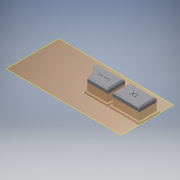
# Autodesk Inventor part: buttons
Saved by Autodesk Inventor 2017.3 (Build 213257000, 257)
## iProperties
Created: 2021-12-05
Part Number: buttons
Material: Generic
Document SubType Name: Modeling
Designer: TEOS
Density: 1 g/cm^3
Appearance: Default
Author: TEOS
Autodesk Inventor part; units mm, degrees
ref_plane "YZ Plane" through (0, 0, 0) normal (1, 0, 0) x (0, 1, 0)
ref_plane "XZ Plane" through (0, 0, 0) normal (0, 1, 0) x (-1, 0, 0)
ref_plane "XY Plane" through (0, 0, 0) normal (0, 0, 1) x (1, 0, 0)
ref_plane "Work Plane1" through (0, 0, 0) normal (0, 0, 1) x (1, 0, 0)
ref_plane "Work Plane2" through (0, 0, 0) normal (0, 0, 1) x (1, 0, 0)
sketch "Sketch3" plane through (0, 0, 0) normal (0, 0, 1) x (1, 0, 0)
  circle A0 centre (67, -22) radius 12.5 projected
  circle A1 centre (27, -22) radius 12.5 projected
  line L0 (-20.5, 34.5) -> (25.5, 34.5) projected
  line L1 (25.5, 34.5) -> (25.5, 4.5) projected
  line L2 (25.5, 4.5) -> (-9.3082, 4.5) projected
  arc A2 (-9.3082, 4.5) -> (-20.5, 25.0657) centre (-48.5, -3.5) ccw projected
  line L3 (-20.5, 25.0657) -> (-20.5, 34.5) projected
  line L4 (79.5, 4.5) -> (33.5, 4.5) projected
  line L5 (33.5, 4.5) -> (33.5, 34.5) projected
  line L6 (33.5, 34.5) -> (79.5, 34.5) projected
  line L7 (79.5, 34.5) -> (79.5, 4.5) projected
  circle A3 centre (-48.5, -3.5) radius 34 projected
  arc A4 (-82, 44) -> (-89, 37) centre (-82, 37) ccw projected
  line L8 (-89, -37) -> (-89, 37) projected
  arc A5 (-89, -37) -> (-82, -44) centre (-82, -37) ccw projected
  line L9 (82, -44) -> (-82, -44) projected
  arc A6 (82, -44) -> (89, -37) centre (82, -37) ccw projected
  line L10 (89, 37) -> (89, -37) projected
  arc A7 (89, 37) -> (82, 44) centre (82, 37) ccw projected
  line L11 (-82, 44) -> (82, 44) projected
  arc A8 (-9.064, 4.8) -> (-20.2, 25.1915) centre (-48.5, -3.5) ccw
  line L12 (-9.064, 4.8) -> (25.2, 4.8)
  line L13 (25.2, 4.8) -> (25.2, 34.2)
  line L14 (25.2, 34.2) -> (-20.2, 34.2)
  line L15 (-20.2, 34.2) -> (-20.2, 25.1915)
  line L16 (33.8, 34.2) -> (33.8, 4.8)
  line L17 (33.8, 4.8) -> (79.2, 4.8)
  line L18 (79.2, 4.8) -> (79.2, 34.2)
  line L19 (79.2, 34.2) -> (33.8, 34.2)
  point P0 (0, 0)
  dimension "d10" = 0.3
  dimension "d11" = 0.3
  constraints: 16 end point, 2 point on circle, 1 centre point, 7 other
  measures "d10" radial gap between concentric circles of A2 A8
  measures "d11" distance between parallel lines of L5 L16
extrude "Extrusion3" add sketch "Sketch3" along normal blind 7 and the other way blind 13 contours A8 L15 L14 L13 L12 | L19 L18 L17 L16
sketch "Sketch4" plane through (0, 0, -13) normal (0, 0, -1) x (-1, 0, 0)
  arc A0 (20.2, 25.1915) -> (9.064, 4.8) centre (48.5, -3.5) ccw projected
  line L0 (20.2, 25.1915) -> (20.2, 34.2) projected
  line L1 (20.2, 34.2) -> (-25.2, 34.2) projected
  line L2 (-25.2, 34.2) -> (-25.2, 4.8) projected
  line L3 (-25.2, 4.8) -> (9.064, 4.8) projected
  line L4 (-33.8, 4.8) -> (-33.8, 34.2) projected
  line L5 (-33.8, 34.2) -> (-79.2, 34.2) projected
  line L6 (-79.2, 34.2) -> (-79.2, 4.8) projected
  line L7 (-79.2, 4.8) -> (-33.8, 4.8) projected
  arc A1 (23.2, 23.908) -> (11.5785, 1.8) centre (48.5, -3.5) ccw
  line L8 (23.2, 23.908) -> (23.2, 37.2)
  line L9 (23.2, 37.2) -> (-28.2, 37.2)
  line L10 (-28.2, 37.2) -> (-28.2, 1.8)
  line L11 (-28.2, 1.8) -> (11.5785, 1.8)
  line L12 (-30.8, 37.2) -> (-30.8, 1.8)
  line L13 (-30.8, 1.8) -> (-82.2, 1.8)
  line L14 (-82.2, 1.8) -> (-82.2, 37.2)
  line L15 (-82.2, 37.2) -> (-30.8, 37.2)
  point P0 (0, 0)
  dimension "d16" = 3
  dimension "d17" = 3
  constraints: 16 end point, 2 point on circle, 1 centre point, 7 other
  measures "d16" radial gap between concentric circles of A0 A1
  measures "d17" distance between parallel lines of L4 L12
extrude "Extrusion4" add sketch "Sketch4" along normal blind 3 contours A0 L3 L2 L1 L0 | L7 L6 L5 L4 | A1 L11 L10 L9 L8 | L12 L13 L14 L15
sketch "Sketch5" plane through (0, 0, -16) normal (0, 0, -1) x (-1, 0, 0)
  arc A0 (23.2, 23.908) -> (11.5785, 1.8) centre (48.5, -3.5) ccw projected
  line L0 (23.2, 23.908) -> (23.2, 37.2) projected
  line L1 (23.2, 37.2) -> (-28.2, 37.2) projected
  line L2 (-28.2, 37.2) -> (-28.2, 1.8) projected
  line L3 (-28.2, 1.8) -> (11.5785, 1.8) projected
  line L4 (-30.8, 1.8) -> (-30.8, 37.2) projected
  line L5 (-30.8, 37.2) -> (-82.2, 37.2) projected
  line L6 (-82.2, 37.2) -> (-82.2, 1.8) projected
  line L7 (-82.2, 1.8) -> (-30.8, 1.8) projected
  line L8 (-82.2, 19.5) -> (15.4079, 19.5) construction
  arc A1 (20.2, 25.1915) -> (9.064, 4.8) centre (48.5, -3.5) ccw construction
  line L9 (-82.2, 37.2) -> (-30.8, 37.2) construction
  line L10 (-56.5, 37.2) -> (-56.5, 1.8) construction
  line L11 (-30.8, 1.8) -> (-82.2, 1.8) construction
  line L12 (23.2, 37.2) -> (-28.2, 37.2) construction
  line L13 (-2.5, 37.2) -> (-2.5, 1.8) construction
  line L14 (-28.2, 1.8) -> (11.5785, 1.8) construction
  point P0 (0, 0)
  point P1 (-16.2, 19.5)
  point P2 (5.2, 19.5)
  point P3 (-70.2, 19.5)
  point P4 (-42.8, 19.5)
  dimension "d20" = 12
  dimension "d21" = 18
  dimension "d22" = 12
  constraints: 6 end point, 5 point on line, 4 midpoint, 1 horizontal, 1 parallel, 1 point on circle, 1 symmetric about line
  measures "d20" distance from line of L2 point (-16.2, 19.5)
  measures "d21" distance from line of L0 point (5.2, 19.5)
  measures "d22" distance from line of L6 point (-70.2, 19.5)
hole "Hole1" at (16.2, 19.5, -16) at (-5.2, 19.5, -16) at (70.2, 19.5, -16) at (42.8, 19.5, -16) direction (0, 0, 1) diameter 5 depth 8
chamfer "Chamfer1" distance 2 angle 45 8 edges at (33.8, 19.5, 7) (56.5, 34.2, 7) (79.2, 19.5, 7) (56.5, 4.8, 7) (2.5, 34.2, 7) (25.2, 19.5, 7) (8.068, 4.8, 7) (-13.1306, 15.8157, 7)
sketch "Sketch6" plane through (0, 0, 7) normal (0, 0, 1) x (1, 0, 0)
  line L0 (62.1554, 16.2385) -> (50.9463, 16.2385) construction
  line L1 (50.9463, 16.2385) -> (50.9463, 23.2385) construction
  line L2 (50.9463, 23.2385) -> (62.1554, 23.2385) construction
  line L3 (62.1554, 23.2385) -> (62.1554, 16.2385) construction
  line L4 (77.2, 32.2) -> (77.2, 6.8) projected
  line L5 (35.8, 6.8) -> (35.8, 32.2) projected
  line L6 (77.2, 6.8) -> (35.8, 32.2)
  line L7 (77.2, 6.8) -> (35.8, 6.8) projected
  line L8 (35.8, 32.2) -> (35.8, 6.8)
  line L9 (35.8, 32.2) -> (77.2, 32.2) projected
  line L10 (35.8, 6.8) -> (77.2, 32.2)
  line L11 (59.8126, 23.2385) -> (59.8126, 17.0667)
  line L12 (59.8126, 17.0667) -> (62.1611, 17.0667)
  line L13 (62.1611, 17.0667) -> (62.1611, 16.2385)
  line L14 (62.1611, 16.2385) -> (56.5338, 16.2385)
  line L15 (56.5338, 16.2385) -> (56.5338, 17.0667)
  line L16 (56.5338, 17.0667) -> (58.8823, 17.0667)
  line L17 (58.8823, 17.0667) -> (58.8823, 23.2385)
  line L18 (58.8823, 23.2385) -> (59.8126, 23.2385)
  line L19 (50.986, 23.2385) -> (52.0525, 23.2385)
  line L20 (52.0525, 23.2385) -> (53.7542, 20.4476)
  line L21 (53.7542, 20.4476) -> (55.4901, 23.2385)
  line L22 (55.4901, 23.2385) -> (56.4941, 23.2385)
  line L23 (56.4941, 23.2385) -> (54.2648, 19.7328)
  line L24 (54.2648, 19.7328) -> (56.426, 16.2385)
  line L25 (56.426, 16.2385) -> (55.3596, 16.2385)
  line L26 (55.3596, 16.2385) -> (53.6919, 18.9784)
  line L27 (53.6919, 18.9784) -> (51.9901, 16.2385)
  line L28 (51.9901, 16.2385) -> (50.986, 16.2385)
  line L29 (50.986, 16.2385) -> (53.1756, 19.6875)
  line L30 (53.1756, 19.6875) -> (50.986, 23.2385)
  point P0 (0, 0)
  constraints: 6 end point, 1 perpendicular, 2 other
emboss "Emboss1" sketch "Sketch6" operation cut depth 25 direction (0, 0, -1) contours L11 L6 L17 L10 | L10 L17 L18 L11 | L14 L15 L16 L17 L6 L11 L12 | L6 L12 L13 L14 | L30 L19 L20 L6 | L6 L20 L21 L23 L24 L10 L26 L27 L28 L29 L30 | L10 L27 L28 | L21 L22 L23 L6 | L24 L25 L26 L10
sketch "Sketch7" plane through (0, 0, 7) normal (0, 0, 1) x (1, 0, 0)
  line L0 (14.8194, 18.056) -> (-5.029, 18.056) construction
  line L1 (-5.029, 18.056) -> (-5.029, 21.7006) construction
  line L2 (-5.029, 21.7006) -> (14.8194, 21.7006) construction
  line L3 (14.8194, 21.7006) -> (14.8194, 18.056) construction
  line L4 (23.2, 6.8) -> (-7.4732, 6.8) projected
  line L5 (-20.2, 32.2) -> (23.2, 32.2) projected
  line L6 (23.2, 6.8) -> (-20.2, 32.2)
  line L7 (23.2, 32.2) -> (23.2, 6.8) projected
  line L8 (-20.2, 32.2) -> (23.2, 32.2)
  line L9 (23.2, 32.2) -> (-20.2, 6.8)
  line L10 (13.648, 21.6269) -> (13.648, 18.541)
  line L11 (13.648, 18.541) -> (14.8223, 18.541)
  line L12 (14.8223, 18.541) -> (14.8223, 18.1269)
  line L13 (14.8223, 18.1269) -> (12.0087, 18.1269)
  line L14 (12.0087, 18.1269) -> (12.0087, 18.541)
  line L15 (12.0087, 18.541) -> (13.1829, 18.541)
  line L16 (13.1829, 18.541) -> (13.1829, 21.6269)
  line L17 (13.1829, 21.6269) -> (13.648, 21.6269)
  line L18 (9.646, 21.6269) -> (10.0885, 21.6269)
  line L19 (10.0885, 21.6269) -> (10.0885, 21.3376)
  spline S0 degree 2 poles (10.0885, 21.3376) (10.2927, 21.5163) (10.6586, 21.7006) (10.8855, 21.7006) knots 0 0 0 1 2 2 2
  spline S1 degree 2 poles (10.8855, 21.7006) (11.0557, 21.7006) (11.3591, 21.5872) (11.4698, 21.4652) knots 0 0 0 1 2 2 2
  spline S2 degree 2 poles (11.4698, 21.4652) (11.5832, 21.3433) (11.708, 20.9717) (11.708, 20.7051) knots 0 0 0 1 2 2 2
  line L20 (11.708, 20.7051) -> (11.708, 19.0005)
  line L21 (11.708, 19.0005) -> (11.2655, 19.0005)
  line L22 (11.2655, 19.0005) -> (11.2655, 20.4981)
  spline S3 degree 2 poles (11.2655, 20.4981) (11.2655, 20.7079) (11.2343, 20.9831) (11.1804, 21.0852) knots 0 0 0 1 2 2 2
  spline S4 degree 2 poles (11.1804, 21.0852) (11.1266, 21.1873) (10.9422, 21.2809) (10.7692, 21.2809) knots 0 0 0 1 2 2 2
  spline S5 degree 2 poles (10.7692, 21.2809) (10.6075, 21.2809) (10.2416, 21.0965) (10.0885, 20.9632) knots 0 0 0 1 2 2 2
  line L23 (10.0885, 20.9632) -> (10.0885, 19.0005)
  line L24 (10.0885, 19.0005) -> (9.646, 19.0005)
  line L25 (9.646, 19.0005) -> (9.646, 21.6269)
  line L26 (6.943, 21.6269) -> (7.3855, 21.6269)
  line L27 (7.3855, 21.6269) -> (7.3855, 20.1293)
  spline S6 degree 2 poles (7.3855, 20.1293) (7.3855, 19.9478) (7.4195, 19.6358) (7.4706, 19.5422) knots 0 0 0 1 2 2 2
  spline S7 degree 2 poles (7.4706, 19.5422) (7.5245, 19.4429) (7.7173, 19.3465) (7.8818, 19.3465) knots 0 0 0 1 2 2 2
  spline S8 degree 2 poles (7.8818, 19.3465) (8.0463, 19.3465) (8.3952, 19.5224) (8.5625, 19.6642) knots 0 0 0 1 2 2 2
  line L28 (8.5625, 19.6642) -> (8.5625, 21.6269)
  line L29 (8.5625, 21.6269) -> (9.005, 21.6269)
  line L30 (9.005, 21.6269) -> (9.005, 19.0005)
  line L31 (9.005, 19.0005) -> (8.5625, 19.0005)
  line L32 (8.5625, 19.0005) -> (8.5625, 19.2926)
  spline S9 degree 2 poles (8.5625, 19.2926) (8.364, 19.1139) (7.9811, 18.9267) (7.7655, 18.9267) knots 0 0 0 1 2 2 2
  spline S10 degree 2 poles (7.7655, 18.9267) (7.3798, 18.9267) (6.943, 19.4373) (6.943, 19.9223) knots 0 0 0 1 2 2 2
  line L33 (6.943, 19.9223) -> (6.943, 21.6269)
  spline S11 degree 2 poles (5.1817, 21.6865) (5.8113, 21.6865) (6.5034, 20.9802) (6.5034, 20.3279) knots 0 0 0 1 2 2 2
  spline S12 degree 2 poles (6.5034, 20.3279) (6.5034, 19.6869) (5.8312, 18.9267) (5.2894, 18.9267) knots 0 0 0 1 2 2 2
  spline S13 degree 2 poles (5.2894, 18.9267) (5.0455, 18.9267) (4.6683, 19.0686) (4.5293, 19.2189) knots 0 0 0 1 2 2 2
  spline S14 degree 2 poles (4.5293, 19.2189) (4.3875, 19.3692) (4.2372, 19.8032) (4.2372, 20.118) knots 0 0 0 1 2 2 2
  line L34 (4.2372, 20.118) -> (4.2372, 20.3591)
  line L35 (4.2372, 20.3591) -> (6.0552, 20.3591)
  spline S15 degree 2 poles (6.0552, 20.3591) (6.0552, 20.8157) (5.5958, 21.3007) (5.1873, 21.3007) knots 0 0 0 1 2 2 2
  spline S16 degree 2 poles (5.1873, 21.3007) (5.0427, 21.3007) (4.7619, 21.2355) (4.6484, 21.1844) knots 0 0 0 1 2 2 2
  spline S17 degree 2 poles (4.6484, 21.1844) (4.5293, 21.1277) (4.3648, 21.0284) (4.3109, 20.9831) knots 0 0 0 1 2 2 2
  line L36 (4.3109, 20.9831) -> (4.2854, 20.9831)
  line L37 (4.2854, 20.9831) -> (4.2854, 21.4652)
  spline S18 degree 2 poles (4.2854, 21.4652) (4.362, 21.4964) (4.5946, 21.5872) (4.6853, 21.6127) knots 0 0 0 1 2 2 2
  spline S19 degree 2 poles (4.6853, 21.6127) (4.8129, 21.6496) (5.0228, 21.6865) (5.1817, 21.6865) knots 0 0 0 1 2 2 2
  spline S20 degree 2 poles (4.6683, 20.0216) (4.674, 19.8429) (4.7477, 19.5819) (4.8186, 19.494) knots 0 0 0 1 2 2 2
  spline S21 degree 2 poles (4.8186, 19.494) (4.8952, 19.3947) (5.1363, 19.2898) (5.315, 19.2898) knots 0 0 0 1 2 2 2
  spline S22 degree 2 poles (5.315, 19.2898) (5.4908, 19.2898) (5.7376, 19.3947) (5.8397, 19.4968) knots 0 0 0 1 2 2 2
  spline S23 degree 2 poles (5.8397, 19.4968) (5.939, 19.6018) (6.0411, 19.8542) (6.0552, 20.0216) knots 0 0 0 1 2 2 2
  line L38 (6.0552, 20.0216) -> (4.6683, 20.0216)
  line L39 (0.2465, 21.6269) -> (0.7882, 21.6269)
  line L40 (0.7882, 21.6269) -> (1.4264, 20.6399)
  line L41 (1.4264, 20.6399) -> (2.0816, 21.6269)
  line L42 (2.0816, 21.6269) -> (2.5836, 21.6269)
  line L43 (2.5836, 21.6269) -> (1.6732, 20.325)
  line L44 (1.6732, 20.325) -> (2.5751, 19.0005)
  line L45 (2.5751, 19.0005) -> (2.0334, 19.0005)
  line L46 (2.0334, 19.0005) -> (1.398, 19.979)
  line L47 (1.398, 19.979) -> (0.7485, 19.0005)
  line L48 (0.7485, 19.0005) -> (0.2465, 19.0005)
  line L49 (0.2465, 19.0005) -> (1.1513, 20.2967)
  line L50 (1.1513, 20.2967) -> (0.2465, 21.6269)
  line L51 (-2.014, 21.6269) -> (-0.3066, 21.6269)
  line L52 (-0.3066, 21.6269) -> (-0.3066, 21.2695)
  line L53 (-0.3066, 21.2695) -> (-0.9419, 21.2695)
  line L54 (-0.9419, 21.2695) -> (-0.9419, 18.9239)
  line L55 (-0.9419, 18.9239) -> (-0.3066, 18.9239)
  line L56 (-0.3066, 18.9239) -> (-0.3066, 18.6034)
  spline S24 degree 2 poles (-0.3066, 18.6034) (-0.6668, 18.6034) (-1.0072, 18.3992) (-1.0298, 18.1156) knots 0 0 0 1 2 2 2
  line L57 (-1.0298, 18.1156) -> (-1.3929, 18.1156)
  line L58 (-1.3929, 18.1156) -> (-1.3929, 21.2695)
  line L59 (-1.3929, 21.2695) -> (-2.014, 21.2695)
  line L60 (-2.014, 21.2695) -> (-2.014, 21.6269)
  spline S25 degree 2 poles (-4.8362, 19.8769) (-4.8362, 20.8186) (-4.2888, 21.7006) (-3.7187, 21.7006) knots 0 0 0 1 2 2 2
  spline S26 degree 2 poles (-3.7187, 21.7006) (-3.1401, 21.7006) (-2.5983, 20.8015) (-2.5983, 19.8797) knots 0 0 0 1 2 2 2
  spline S27 degree 2 poles (-2.5983, 19.8797) (-2.5983, 18.9324) (-3.1457, 18.056) (-3.7187, 18.056) knots 0 0 0 1 2 2 2
  spline S28 degree 2 poles (-3.7187, 18.056) (-4.2944, 18.056) (-4.8362, 18.9636) (-4.8362, 19.8769) knots 0 0 0 1 2 2 2
  spline S29 degree 2 poles (-4.2349, 20.9434) (-4.3029, 20.7703) (-4.3597, 20.2371) (-4.3597, 19.8769) knots 0 0 0 1 2 2 2
  spline S30 degree 2 poles (-4.3597, 19.8769) (-4.3597, 19.5167) (-4.3029, 18.9863) (-4.232, 18.8076) knots 0 0 0 1 2 2 2
  spline S31 degree 2 poles (-4.232, 18.8076) (-4.1611, 18.6289) (-3.9144, 18.4446) (-3.7187, 18.4446) knots 0 0 0 1 2 2 2
  spline S32 degree 2 poles (-3.7187, 18.4446) (-3.523, 18.4446) (-3.2705, 18.6289) (-3.1968, 18.8133) knots 0 0 0 1 2 2 2
  spline S33 degree 2 poles (-3.1968, 18.8133) (-3.1259, 18.992) (-3.0748, 19.5365) (-3.0748, 19.8797) knots 0 0 0 1 2 2 2
  spline S34 degree 2 poles (-3.0748, 19.8797) (-3.0748, 20.2485) (-3.1202, 20.742) (-3.1939, 20.9348) knots 0 0 0 1 2 2 2
  spline S35 degree 2 poles (-3.1939, 20.9348) (-3.262, 21.1164) (-3.5144, 21.3121) (-3.7187, 21.3121) knots 0 0 0 1 2 2 2
  spline S36 degree 2 poles (-3.7187, 21.3121) (-3.9115, 21.3121) (-4.164, 21.1277) (-4.2349, 20.9434) knots 0 0 0 1 2 2 2
  point P0 (0, 0)
  constraints: 6 end point, 1 perpendicular, 2 other
emboss "Emboss2" sketch "Sketch7" operation cut depth 30 direction (0, 0, -1) contours L60 L51 L52 L53 L54 L6 L58 L59 | L6 L59 L60 | S11 S12 S13 S14 L34 L35 S15 S16 S17 L36 L37 L9 | L9 L37 S18 S19 S11 | L45 L46 L6 | L6 L46 L9 L44 L45 | L6 L54 L55 L56 S24 L57 L58 | L9 L46 L47 L6 L49 L50 L39 L40 L41 L42 L43 L44 | L6 L47 L9 L48 L49 | L47 L48 L9 | L10 L11 L12 L13 L14 L15 L16 L17 | L18 L19 S0 S1 S2 L20 L21 L22 S3 S4 S5 L23 L24 L25 | L26 L27 S6 S7 S8 L28 L29 L30 L31 L32 S9 S10 L33 | S25 S26 S27 S28
body "Solid2"
